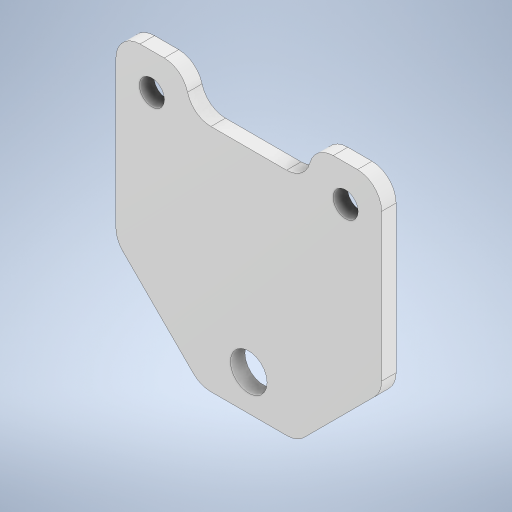
# Autodesk Inventor part: Gantry Plate
Saved by Autodesk Inventor 2023 (Build 270158000, 158)
## iProperties
Created: 2023-04-10
Part Number: Gantry Plate
Material: PC/ABS Plastic
Document SubType Name: Modeling
Designer: ethan
Density: 0.357273 g/cm^3
Appearance: Smooth - White
Author: ethan
Autodesk Inventor part; units mm, degrees
ref_plane "YZ Plane" through (0, 0, 0) normal (1, 0, 0) x (0, 1, 0)
ref_plane "XZ Plane" through (0, 0, 0) normal (0, 1, 0) x (-1, 0, 0)
ref_plane "XY Plane" through (0, 0, 0) normal (0, 0, 1) x (1, 0, 0)
sketch "Sketch1" plane through (0, 0, 0) normal (0, 1, 0) x (-1, 0, 0)
  line L0 (0, 0) -> (55, 0)
  line L1 (55, 0) -> (55, -55)
  line L2 (55, -55) -> (0, -55)
  line L3 (0, -55) -> (0, 0)
  line L4 (47.55, -7.45) -> (7.45, -7.45) construction
  line L5 (7.45, -7.45) -> (7.45, -47.55) construction
  line L6 (7.45, -47.55) -> (47.55, -47.55) construction
  line L7 (47.55, -47.55) -> (47.55, -7.45) construction
  circle A0 centre (47.55, -47.55) radius 2.6
  circle A1 centre (7.45, -47.55) radius 2.6
  circle A2 centre (27.5, -7.45) radius 3.8
  line L8 (0, -17.5) -> (17.5, 0)
  line L9 (37.5, 0) -> (55, -17.5)
  line L10 (17.5, -55) -> (37.5, -55)
  line L11 (15, -55) -> (40, -55)
  line L12 (40, -55) -> (40, -47.55)
  line L13 (40, -47.55) -> (15, -47.55)
  line L14 (15, -47.55) -> (15, -55)
  dimension "d0" = 55
  dimension "d1" = 55
  dimension "d2" = 40.1
  dimension "d3" = 40.1
  dimension "d6" = 5.2
  dimension "d7" = 5.2
  dimension "d8" = 7.45
  dimension "d9" = 7.45
  dimension "d14" = 7.6
  dimension "d55" = 20
  dimension "d56" = 10
  dimension "d87" = 15
  dimension "d88" = 15
  constraints: 30 end point, 7 point on line, 6 parallel, 5 perpendicular, 4 horizontal, 3 centre point, 2 coincident, 1 midpoint
  measures "d0" distance of L1.end L2.end
  measures "d1" distance of L0.end L1.end
  measures "d2" distance of L6.end L5.end
  measures "d3" distance of L5.end L4.end
  measures "d6" diameter of A0
  measures "d7" diameter of A1
  measures "d8" distance between parallel lines of L1 L7
  measures "d9" distance from line of L2 L5.end
  measures "d14" diameter of A2
  measures "d55" distance of L9.start L8.end
  measures "d56" horizontal distance of L8.end A2.centre
  measures "d87" distance between parallel lines of L3 L14
  measures "d88" distance between parallel lines of L1 L12
extrude "Extrusion1" add sketch "Sketch1" along normal blind 3 contours L0 L9 L1 L2 L12 L13 L14 L3 L8
fillet "Fillet1" radius 5 10 edges at (-55, 1.5, -55) (0, 1.5, -55) (-55, 1.5, -17.5) (-37.5, 1.5, 0) (-17.5, 1.5, 0) (0, 1.5, -17.5) (-15, 1.5, -55) (-40, 1.5, -55) (-15, 1.5, -47.55) (-40, 1.5, -47.55)
equation "\"d1\" = d0"
equation "\"d3\" = d2"
equation "\"d8\" = -0.5 * d2 + 0.5 * d0"
equation "\"d9\" = -0.5 * d3 + 0.5 * d1"
equation "\"d88\" = d87"
body "Solid1"
